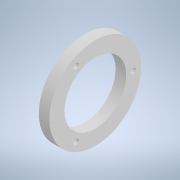
# Autodesk Inventor part: Soporte2_Rodamientos
Saved by Autodesk Inventor 2020.1 (Build 241239000, 239)
## iProperties
Created: 2019-12-08
Part Number: Soporte2_Rodamientos
Material: Generic
Document SubType Name: Modeling
Designer: Daniel
Density: 1 g/cm^3
Appearance: Default
Author: Daniel
Autodesk Inventor part; units mm, degrees
ref_plane "YZ Plane" through (0, 0, 0) normal (1, 0, 0) x (0, 1, 0)
ref_plane "XZ Plane" through (0, 0, 0) normal (0, 1, 0) x (-1, 0, 0)
ref_plane "XY Plane" through (0, 0, 0) normal (0, 0, 1) x (1, 0, 0)
sketch "Sketch1" plane through (0, 0, 0) normal (1, 0, 0) x (0, 1, 0)
  circle A0 centre (0, 0) radius 26
  circle A1 centre (0, 0) radius 17.5
  line L0 (9.2645, 0) -> (-12.3906, 0) construction
  circle A2 centre (0, 0) radius 21.5 construction
  line L1 (0, 0) -> (0, -36.6713) construction
  point P0 (0, -21.5)
  point P1 (18.6195, 10.75)
  point P2 (-18.6195, 10.75)
  dimension "d1" = 43
  dimension "d0" = 35
  dimension "d2" = 52
  dimension "d5" = 360
  constraints: 4 end point, 3 coincident, 2 centre point, 2 horizontal, 1 point on line, 1 vertical, 1 vertical alignment, 9 other
  measures "d0" diameter of A1
  measures "d2" diameter of A0
extrude "Extrusion1" add sketch "Sketch1" along normal blind 6
hole "Hole1" at (0, 0, -21.5) at (0, 18.6195, 10.75) at (0, -18.6195, 10.75) direction (1, 0, 0) diameter 3 depth 10 tip angle 118
body "Solid1"
